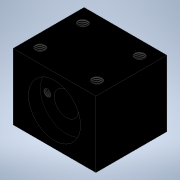
# Autodesk Inventor part: AoVitmeT8
Saved by Autodesk Inventor 2020 (Build 240168000, 168)
## iProperties
Created: 2020-03-25
Part Number: AoVitmeT8
Material: Generic
Document SubType Name: Modeling
Designer: Personal Computer
Density: 1 g/cm^3
Appearance: Anodized - Black
Author: Personal Computer
Autodesk Inventor part; units mm, degrees
ref_plane "YZ Plane" through (0, 0, 0) normal (1, 0, 0) x (0, 1, 0)
ref_plane "XZ Plane" through (0, 0, 0) normal (0, 1, 0) x (-1, 0, 0)
ref_plane "XY Plane" through (0, 0, 0) normal (0, 0, 1) x (1, 0, 0)
sketch "Sketch1" plane through (0, 0, 0) normal (0, 0, 1) x (1, 0, 0)
  line L0 (0, 0) -> (17.5, 0)
  line L1 (17.5, 0) -> (17.5, 28)
  line L2 (17.5, 28) -> (-17.5, 28)
  line L3 (-17.5, 28) -> (-17.5, 0)
  line L4 (-17.5, 0) -> (17.5, 0)
  dimension "d0" = 17.5
  dimension "d1" = 28
  dimension "d2" = 35
  constraints: 10 end point, 4 perpendicular, 1 horizontal, 1 point on line
  measures "d0" distance of L0.start L0.end
  measures "d1" distance of L0.end L1.end
  measures "d2" distance of L1.end L2.end
extrude "Extrusion1" add sketch "Sketch1" along normal blind 30
sketch "Sketch2" plane through (0, 0, 30) normal (0, 0, 1) x (1, 0, 0)
  circle A0 centre (0, 14) radius 5.1
  line L0 (17.5, 28) -> (-17.5, 28) projected
  line L1 (-17.5, 28) -> (-17.5, 0) projected
  point P0 (0, 0)
  dimension "d5" = 10.2
  dimension "d6" = 14
  dimension "d85" = 17.5
  constraints: 1 centre point
  measures "d5" diameter of A0
  measures "d6" distance from line of A0.centre L0
  measures "d85" distance from line of L1 A0.centre
extrude "Extrusion2" cut sketch "Sketch2" against normal blind 30
sketch "Sketch4" plane through (-17.5, 28, 0) normal (0, 1, 0) x (1, 0, 0)
  line L0 (0, -30) -> (35, -30) projected
  line L1 (17.5, -30) -> (17.5, 3.7121)
  line L2 (0, 0) -> (0, -30) projected
  circle A0 centre (29.5, -6) radius 2
  circle A1 centre (5.5, -6) radius 2
  line L3 (34, -15) -> (-3.2563, -15)
  line L4 (35, 0) -> (0, 0) projected
  circle A2 centre (29.5, -24) radius 2
  circle A3 centre (5.5, -24) radius 2
  line L5 (35, 0) -> (35, -30) projected
  dimension "d37" = 17.5
  dimension "d38" = 4
  dimension "d39" = 4
  dimension "d42" = 15
  dimension "d43" = 4
  dimension "d44" = 4
  dimension "d61" = 6
  dimension "d62" = 6
  dimension "d63" = 6
  dimension "d64" = 6
  dimension "d86" = 12
  dimension "d87" = 12
  dimension "d88" = 12
  dimension "d89" = 12
  constraints: 4 centre point, 4 end point, 1 horizontal, 1 midpoint, 1 perpendicular
  measures "d37" distance between parallel lines of L2 L1
  measures "d38" diameter of A0
  measures "d39" diameter of A1
  measures "d42" distance between parallel lines of L4 L3
  measures "d43" diameter of A2
  measures "d44" diameter of A3
  measures "d61" distance from line of L4 A0.centre
  measures "d62" distance from line of A1.centre L4
  measures "d63" distance from line of L0 A3.centre
  measures "d64" distance from line of L0 A2.centre
  measures "d86" distance from line of A1.centre L1
  measures "d87" distance from line of A3.centre L1
  measures "d88" distance from line of L1 A0.centre
  measures "d89" distance from line of L1 A2.centre
extrude "Extrusion4" cut sketch "Sketch4" against normal blind 10 contours A0 | A1 | A2 | A3
thread "Thread7" size "M4x0.7" class "6H" standard "ANSI Metric M Profile" length 10
thread "Thread8" size "M4x0.7" class "6H" standard "ANSI Metric M Profile" full length
thread "Thread9" size "M4x0.7" class "6H" standard "ANSI Metric M Profile" length 10
thread "Thread10" size "M4x0.7" class "6H" standard "ANSI Metric M Profile" length 10
sketch "Sketch7" plane through (0, 0, 30) normal (0, 0, 1) x (1, 0, 0)
  circle A0 centre (0, 14) radius 5.1 projected
  circle A1 centre (0, 14) radius 11
  point P0 (0, 0)
  dimension "d72" = 22
  constraints: 1 centre point, 1 coincident
  measures "d72" diameter of A1
extrude "Extrusion5" cut sketch "Sketch7" against normal blind 5
sketch "Sketch9" plane through (0, 14, 25) normal (0, 0, 1) x (1, 0, 0)
  circle A0 centre (-8, 0) radius 1.5
  circle A1 centre (8, 0) radius 1.5
  point P0 (0, -14)
  dimension "d76" = 3
  dimension "d78" = 3
  constraints: 2 centre point
  measures "d76" diameter of A0
  measures "d78" diameter of A1
extrude "Extrusion6" cut sketch "Sketch9" against normal blind 10
thread "Thread11" size "M3x0.5" class "6H" standard "ANSI Metric M Profile" length 10
thread "Thread12" size "M3x0.5" class "6H" standard "ANSI Metric M Profile" length 10
body "Solid1"
